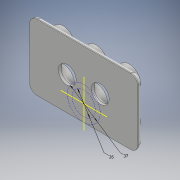
# Autodesk Inventor part: NespressoSpeedfiller-6X-long-tamper
Saved by Autodesk Inventor 2017 (Build 210142000, 142)
## iProperties
Created: 2018-08-27
Part Number: NespressoSpeedfiller-6X-long-tamper
Material: Generic
Document SubType Name: Modeling
Designer: 45027374
Density: 1 g/cm^3
Appearance: Default
Author: 45027374
Autodesk Inventor part; units mm, degrees
ref_plane "YZ Plane" through (0, 0, 0) normal (1, 0, 0) x (0, 1, 0)
ref_plane "XZ Plane" through (0, 0, 0) normal (0, 1, 0) x (-1, 0, 0)
ref_plane "XY Plane" through (0, 0, 0) normal (0, 0, 1) x (1, 0, 0)
sketch "Sketch1" plane through (0, 0, 0) normal (0, 1, 0) x (-1, 0, 0)
  line L0 (25.9, 0) -> (-25.9, 0) projected
  line L1 (0, -25.9) -> (0, 25.9) projected
  circle A0 centre (0, 0) radius 18.5 construction
  circle A1 centre (0, 0) radius 13 construction
  dimension "d0" = 37
  dimension "d1" = 26
  constraints: 2 centre point, 2 coincident
  measures "d0" diameter of A0
  measures "d1" diameter of A1
sketch "Sketch2" plane through (0, 0, 0) normal (0, 1, 0) x (-1, 0, 0)
  line L0 (84.7, 0) -> (-84.7, 0) projected
  line L1 (0, -33.3) -> (0, 70.3) projected
  line L2 (-60.5, 55.5) -> (-60.5, -18.5)
  line L3 (-60.5, -18.5) -> (60.5, -18.5)
  line L4 (60.5, -18.5) -> (60.5, 55.5)
  line L5 (-60.5, 55.5) -> (60.5, 55.5)
  circle A0 centre (0, 37) radius 18.5 construction
  point P0 (0, 0)
  dimension "d3" = 121
  dimension "d29" = 18.5
  dimension "d30" = 55.5
  dimension "d99" = 37
  dimension "d100" = 37
  constraints: 8 end point, 1 centre point, 1 horizontal, 1 parallel, 1 point on line, 1 other
  measures "d3" distance of L2.end L3.end
  measures "d29" distance between parallel lines of L0 L3
  measures "d30" distance between parallel lines of L5 L0
  measures "d99" diameter of A0
  measures "d100" distance of point (0, 0) A0.centre
extrude "Extrusion1" add sketch "Sketch2" along normal blind 6
sketch "Sketch6" plane through (0, 0, 0) normal (0, 1, 0) x (-1, 0, 0)
  line L0 (60.5, -18.5) -> (-60.5, -18.5) projected
  line L1 (60.5, 55.5) -> (60.5, -18.5) projected
  line L2 (-60.5, -18.5) -> (60.5, -18.5)
  line L3 (60.5, -18.5) -> (60.5, 55.5)
  line L4 (-60.5, 55.5) -> (-60.5, -18.5)
  line L5 (84.7, 0) -> (-84.7, 0) projected
  line L6 (0, -36.3) -> (0, 70.8) projected
  arc A0 (-16, 0) -> (16, 0) centre (0, 0) ccw
  line L7 (16, 0) -> (16, 55.5)
  line L8 (60.5, 55.5) -> (-60.5, 55.5) projected
  line L9 (16, 55.5) -> (60.5, 55.5)
  line L10 (-16, 0) -> (-16, 55.5)
  line L11 (-16, 55.5) -> (-60.5, 55.5)
  point P0 (-17.3617, -21)
  dimension "d18" = 32
  constraints: 14 end point, 3 perpendicular, 3 point on line, 2 point on circle, 1 centre point, 1 coincident, 1 collinear, 1 horizontal, 1 parallel, 1 vertical, 1 other
  measures "d18" diameter of A0
extrude "Extrusion5" [suppressed]
sketch "Sketch4" plane through (0, 0, 0) normal (0, 0, 1) x (1, 0, 0)
  line L0 (-18.5, 0) -> (18.5, 0)
  line L1 (18.5, 0) -> (18.5, -2)
  line L2 (18.5, -2) -> (-18.5, -2)
  line L3 (-18.5, -2) -> (-18.5, 0)
  line L4 (-25.9, 0) -> (25.9, 0) projected
  line L5 (0, -2.4) -> (0, 0.4) projected
  point P0 (0, 0)
  dimension "d10" = 37
  dimension "d11" = 2
  constraints: 8 end point, 2 parallel, 1 collinear, 1 horizontal, 1 perpendicular, 1 other
  measures "d10" distance between parallel lines of L1 L3
  measures "d11" distance of L0.end L1.end
extrude "Extrusion6" [suppressed]
sketch "Sketch5" plane through (0, 0, 0) normal (0, 1, 0) x (-1, 0, 0)
  circle A0 centre (0, 0) radius 18.5 construction
  circle A1 centre (0, 0) radius 18.5 construction
  line L0 (25.9, 0) -> (-25.9, 0) projected
  line L1 (0, -28.9) -> (0, 26.4) projected
  line L2 (-18.5, -21) -> (18.5, -21)
  line L3 (18.5, -21) -> (18.5, -18.5)
  line L4 (18.5, -18.5) -> (-18.5, -18.5)
  line L5 (-18.5, -18.5) -> (-18.5, -21)
  dimension "d25" = 37
  dimension "d26" = 21
  constraints: 8 end point, 2 parallel, 1 centre point, 1 coincident, 1 concentric, 1 horizontal, 1 perpendicular, 1 tangent, 1 other
  measures "d25" distance of L2.start L2.end
  measures "d26" distance between parallel lines of L0 L2
extrude "Extrusion7" [suppressed]
sketch "Sketch7" plane through (0, 0, 0) normal (0, 0, 1) x (1, 0, 0)
  line L0 (-18.5, 0) -> (18.5, 0)
  line L1 (18.5, 0) -> (18.5, -2)
  line L2 (18.5, -2) -> (-18.5, -2)
  line L3 (-18.5, -2) -> (-18.5, 0)
  line L4 (60.5, 0) -> (-60.5, 0) projected
  line L5 (-84.7, 0) -> (84.7, 0) projected
  line L6 (0, -2.4) -> (0, 0.4) projected
  point P0 (-16, 0)
  point P1 (16, 0)
  dimension "d53" = 2
  dimension "d54" = 18.5
  constraints: 8 end point, 2 parallel, 1 collinear, 1 horizontal, 1 perpendicular, 1 other
  measures "d53" distance of L0.end L1.end
  measures "d54" distance between parallel lines of L6 L1
extrude "Extrusion8" [suppressed]
sketch "Sketch8" plane through (0, 0, 0) normal (0, 1, 0) x (-1, 0, 0)
  circle A0 centre (0, 0) radius 12.75
  dimension "d34" = 25.5
  constraints: 1 centre point, 1 coincident
  measures "d34" diameter of A0
extrude "Extrusion9" add sketch "Sketch8" along normal blind 14
pattern_linear "Rectangular Pattern1" count 2 spacing 37 along (0, 0, 1) count 3 spacing 37 along (1, 0, 0) of "Extrusion9" second direction both ways yes
sketch "Sketch9" plane through (0, 6, 0) normal (0, 1, 0) x (1, 0, 0)
  circle A0 centre (0, 0) radius 13
  circle A1 centre (0, 0) radius 15
  dimension "d40" = 26
  dimension "d41" = 30
  constraints: 2 centre point, 2 coincident
  measures "d40" diameter of A0
  measures "d41" diameter of A1
extrude "Extrusion10" [suppressed]
sketch "Sketch10" plane through (0, 5, 0) normal (0, 1, 0) x (1, 0, 0)
  arc A0 (16, 0) -> (-16, 0) centre (0, 0) ccw projected
  line L0 (1.5, -18) -> (-1.5, -18)
  line L1 (-29.4, 0) -> (29.4, 0) projected
  line L2 (0, 36.3) -> (0, -70.8) projected
  line L3 (1.5, -12) -> (-1.5, -12)
  line L4 (1.5, -12) -> (1.5, -18)
  line L5 (-1.5, -18) -> (-1.5, -12)
  dimension "d48" = 3
  dimension "d49" = 12
  dimension "d50" = 6
  constraints: 8 end point, 2 perpendicular, 1 horizontal, 1 parallel, 1 other
  measures "d48" distance between parallel lines of L4 L5
  measures "d49" distance between parallel lines of L1 L3
  measures "d50" distance between parallel lines of L0 L3
extrude "Extrusion11" [suppressed]
fillet "Fillet1" [suppressed]
sketch "Sketch11" plane through (0, 0, 0) normal (0, 1, 0) x (-1, 0, 0)
  line L0 (-60.5, -21) -> (60.5, -21)
  line L1 (60.5, -21) -> (60.5, -47)
  line L2 (60.5, -47) -> (-60.5, -47)
  line L3 (-60.5, -47) -> (-60.5, -21)
  line L4 (84.7, 0) -> (-84.7, 0) projected
  line L5 (0, -60.1) -> (0, 31.6) projected
  point P0 (0, 0)
  dimension "d57" = 26
  dimension "d58" = 21
  dimension "d59" = 121
  constraints: 8 end point, 2 parallel, 1 horizontal, 1 perpendicular, 1 other
  measures "d57" distance of L0.end L1.end
  measures "d58" distance between parallel lines of L4 L0
  measures "d59" distance between parallel lines of L1 L3
extrude "Extrusion12" [suppressed]
sketch "Sketch12" plane through (0, 0, 0) normal (1, 0, 0) x (0, 1, 0)
  line L0 (6, 55.5) -> (6, -18.5) projected
  arc A0 (6, -16.5081) -> (5.7334, -47) centre (34, -32) ccw
  line L1 (-6.8, 0) -> (40.8, 0) projected
  line L2 (0, -67.5) -> (0, 76) projected
  line L3 (6, -16.5081) -> (6, -47)
  line L4 (6, -47) -> (5.7334, -47)
  line L5 (0, -47) -> (6, -47) projected
  point P0 (0, 0)
  point P1 (6, 48)
  dimension "d62" = 32
  dimension "d63" = 32
  dimension "d64" = 34
  constraints: 4 end point, 2 point on circle, 2 point on line, 1 centre point, 1 collinear
  measures "d62" radius of A0
  measures "d63" distance from line of L1 A0.centre
  measures "d64" distance from line of A0.centre L2
extrude "Extrusion13" [suppressed]
fillet "Fillet3" [suppressed]
sketch "Sketch13" plane through (0, 0, 0) normal (0, 1, 0) x (-1, 0, 0)
  line L0 (84.7, 0) -> (-84.7, 0) projected
  line L1 (0, -67.5) -> (0, 76) projected
  line L2 (60.5, 55.5) -> (60.5, -18.5) projected
  arc A0 (13.0815, 23.9185) -> (13.0815, 13.0815) centre (18.5, 18.5) ccw
  line L3 (-60.5, 55.5) -> (-60.5, -18.5) projected
  arc A1 (-13.0815, 13.0815) -> (-13.0815, 23.9185) centre (-18.5, 18.5) ccw
  line L4 (18.5, 37) -> (18.5, 0)
  line L5 (-18.5, 0) -> (-18.5, 37)
  line L6 (18.5, 37) -> (18.5, 55.5)
  line L7 (-60.5, 55.5) -> (60.5, 55.5) projected
  line L8 (-18.5, 55.5) -> (-18.5, 37)
  arc A2 (-9.2871, 53) -> (-13.0815, 23.9185) centre (0, 37) ccw
  arc A3 (13.0815, 23.9185) -> (9.2871, 53) centre (0, 37) ccw
  arc A4 (-13.0815, 13.0815) -> (-18.5, 0) centre (0, 0) ccw
  arc A5 (18.5, 0) -> (13.0815, 13.0815) centre (0, 0) ccw
  point P0 (60.5, -39.254)
  point P1 (-55.5, 48)
  point P2 (-60.5, -16.5081)
  point P3 (-60.5, -47)
  point P4 (60.5, -18.5)
  point P5 (-60.5, -18.5)
  dimension "d68" = 37
  dimension "d71" = 18.5
  dimension "d72" = 18.5
  dimension "d73" = 7.663
  dimension "d74" = 7.663
  dimension "d75" = 18.5
  dimension "d76" = 18.5
  dimension "d77" = 18.5
  dimension "d78" = 18.5
  constraints: 14 point on circle, 8 end point, 6 centre point, 1 coincident, 1 parallel, 1 point on line, 1 vertical, 11 other
  measures "d68" distance of A2.centre point (0, 0)
  measures "d71" radius of A5
  measures "d72" radius of A4
  measures "d73" radius of A0
  measures "d74" radius of A1
  measures "d75" radius of A2
  measures "d76" radius of A3
  measures "d77" distance from line of L0 A0.centre
  measures "d78" distance from line of L0 A1.centre
extrude "Extrusion14" [suppressed]
sketch "Sketch14" plane through (0, 0, 0) normal (0, 1, 0) x (-1, 0, 0)
  circle A0 centre (18.5, 18.5) radius 10
  line L0 (39.9, 0) -> (-39.9, 0) projected
  line L1 (0, -27.9) -> (0, 37.9) projected
  circle A1 centre (-18.5, 18.5) radius 10
  point P0 (0, 0)
  dimension "d84" = 18.5
  dimension "d85" = 18.5
  dimension "d86" = 20
  dimension "d89" = 37
  constraints: 2 centre point, 1 horizontal, 2 other
  measures "d84" distance from line of L0 A0.centre
  measures "d85" distance from line of L1 A0.centre
  measures "d86" diameter of A0
  measures "d89" distance of A0.centre A1.centre
extrude "Extrusion15" cut sketch "Sketch14" along normal through all
fillet "Fillet4" radius 3 2 edges at (-8.5, 6, 18.5) (28.5, 6, 18.5)
fillet "Fillet5" radius 8 4 edges at (-60.5, 3, 55.5) (60.5, 3, 55.5) (-60.5, 3, -18.5) (60.5, 3, -18.5)
fillet "Fillet6" radius 5 5 edges at (58.1569, 6, 53.1569) (60.5, 6, 18.5) (-58.1569, 6, 53.1569) (-60.5, 6, 18.5) (0, 6, 55.5)
equation "\"d85\" = d84"
body "Solid1"
